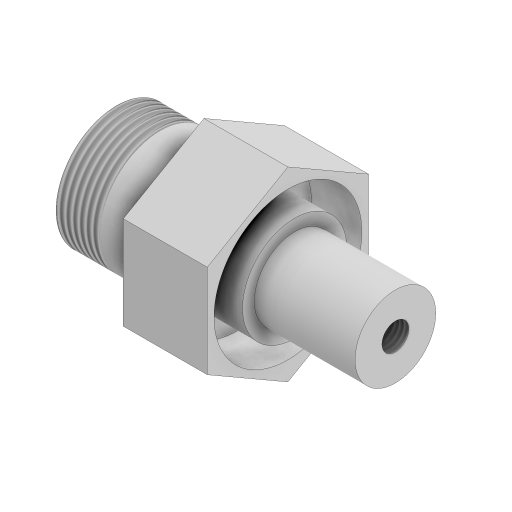
# Autodesk Inventor part: HEX HUB ver 1
Saved by Autodesk Inventor 2023 (Build 270158000, 158)
## iProperties
Created: 2023-03-21
Part Number: HEX HUB ver 1
Material: Generic
Document SubType Name: Modeling
Designer: Juyoung Han
Density: 1 g/cm^3
Appearance: Default
Mass: 7.90916 g
Surface Area: 51.3372 cm^2
Volume: 7.90916 cm^3
Author: Juyoung Han
Autodesk Inventor part; units mm, degrees
ref_plane "YZ Plane" through (0, 0, 0) normal (1, 0, 0) x (0, 1, 0)
ref_plane "XZ Plane" through (0, 0, 0) normal (0, 1, 0) x (-1, 0, 0)
ref_plane "XY Plane" through (0, 0, 0) normal (0, 0, 1) x (1, 0, 0)
sketch "Sketch1" plane through (0, 0, 0) normal (0, 0, 1) x (1, 0, 0)
  line L0 (0, 0) -> (-13, 0)
  line L1 (-13, 0) -> (-13, 9)
  line L2 (-13, 9) -> (0, 9)
  line L3 (0, 9) -> (0, 12)
  line L4 (0, 12) -> (12.5, 12)
  line L5 (12.5, 12) -> (12.5, 11)
  line L6 (12.5, 11) -> (5, 11)
  line L7 (5, 11) -> (5, 7.75)
  line L8 (5, 7.75) -> (13.5, 7.75)
  line L9 (13.5, 7.75) -> (13.5, 6)
  line L10 (13.5, 6) -> (28.5, 6)
  line L11 (28.5, 6) -> (28.5, 0)
  line L12 (28.5, 0) -> (0, 0)
  dimension "d0" = 13
  dimension "d1" = 9
  dimension "d2" = 13
  dimension "d3" = 3
  dimension "d4" = 12.5
  dimension "d5" = 1
  dimension "d6" = 7.5
  dimension "d7" = 3.25
  dimension "d8" = 8.5
  dimension "d9" = 1.75
  dimension "d10" = 15
  constraints: 26 end point, 11 perpendicular, 2 horizontal
  measures "d0" distance of L0.start L0.end
  measures "d1" distance of L0.end L1.end
  measures "d2" distance of L1.end L2.end
  measures "d3" distance of L2.end L3.end
  measures "d4" distance of L3.end L4.end
  measures "d5" distance of L4.end L5.end
  measures "d6" distance of L5.end L6.end
  measures "d7" distance of L6.end L7.end
  measures "d8" distance of L7.end L8.end
  measures "d9" distance of L8.end L9.end
  measures "d10" distance of L9.end L10.end
revolve "Revolution1" add sketch "Sketch1" angle 360 about axis through (28.5, 0, 0) along (-1, 0, 0)
sketch "Sketch2" plane through (12.5, 0, 0) normal (1, 0, 0) x (0, 0, -1)
  circle A0 centre (0, 0) radius 12 projected
  line L0 (12, -6.9282) -> (0, -13.8564)
  line L1 (0, -13.8564) -> (-12, -6.9282)
  line L2 (-12, -6.9282) -> (-12, 6.9282)
  line L3 (-12, 6.9282) -> (0, 13.8564)
  line L4 (0, 13.8564) -> (12, 6.9282)
  line L5 (12, 6.9282) -> (12, -6.9282)
  circle A1 centre (0, 0) radius 11
  point P0 (12, 0)
  point P1 (6, 10.3923)
  point P2 (6, -10.3923)
  point P3 (-6, 10.3923)
  point P4 (-12, 0)
  point P5 (-6, -10.3923)
  dimension "d12" = 24
  dimension "d13" = 0
  constraints: 12 end point, 2 coincident, 1 centre point, 13 other
  measures "d12" distance between parallel lines of L4 L1
  measures "d13" horizontal distance of point (0, 0) L3.end
extrude "Extrusion1" add sketch "Sketch2" against normal blind 12.5 contours L5 L0 A0 | A0 L4 L5 | A0 L3 L4 | L0 L1 A0 | A0 L2 L3 | L1 L2 A0
thread "Thread1" size "M18x1" class "6g" standard "ANSI Metric M Profile" length 7 offset 6.5
sketch "Sketch3" plane through (-13, 0, 0) normal (-1, 0, 0) x (0, 0, 1)
  circle A0 centre (0, 0) radius 7.75 projected
  circle A1 centre (0, 0) radius 6.5
  dimension "d18" = 13
  constraints: 1 centre point, 1 coincident
  measures "d18" diameter of A1
extrude "Extrusion2" cut sketch "Sketch3" against normal blind 13 contours A1
sketch "Sketch4" plane through (0, 0, 0) normal (-1, 0, 0) x (0, 0, 1)
  circle A0 centre (0, 0) radius 2
  dimension "d21" = 4
  constraints: 1 centre point, 1 coincident
  measures "d21" diameter of A0
extrude "Extrusion3" cut sketch "Sketch4" against normal through all
thread "Thread2" size "M4x0.7" class "6H" standard "ANSI Metric M Profile" length 28.5
body "Solid1"
